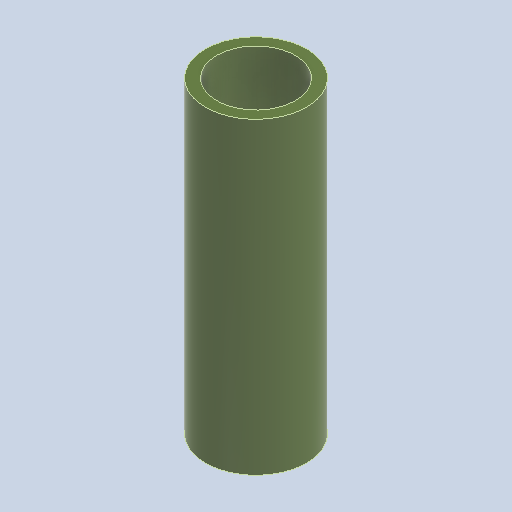
# Autodesk Inventor part: rotor_sleeve
Saved by Autodesk Inventor 2025 (Build 290162000, 162)
## iProperties
Created: 2026-08-13
Part Number: rotor_sleeve
Material: Ogólny
Document SubType Name: Modeling
Designer: zzapa
Density: 1 g/cm^3
Appearance: Ciemnooliwkowa
Author: zzapa
Autodesk Inventor part; units mm, degrees
ref_plane "YZ Plane" through (0, 0, 0) normal (1, 0, 0) x (0, 1, 0)
ref_plane "XZ Plane" through (0, 0, 0) normal (0, 1, 0) x (-1, 0, 0)
ref_plane "XY Plane" through (0, 0, 0) normal (0, 0, 1) x (1, 0, 0)
sketch "Szkic1" plane through (0, 0, 0) normal (0, 1, 0) x (-1, 0, 0)
  circle A0 centre (0, 0) radius 5.25
  circle A1 centre (0, 0) radius 4.075
  dimension "d0" = 8.15
  dimension "d1" = 10.5
  constraints: 2 centre point, 2 coincident
  measures "d0" diameter of A1
  measures "d1" diameter of A0
extrude "Wyciągnięcie proste1" add sketch "Szkic1" along normal blind 32
equation "\"d0\" = rotor_sleeve_in_D"
equation "\"d1\" = rotor_sleeve_out_D"
equation "\"d2\" = rotor_sleeve_h"
equation "\"insert_m2_d\" = 2.9"
equation "\"insert_m2_h\" = 7"
equation "\"insert_m2_corner\" = 0.5"
equation "\"insert_m2_pocket_d\" = 2.6"
equation "\"insert_m2_pocket_D\" = 4.5"
equation "\"insert_m2_pocket_nut_h\" = 1.5"
equation "\"stator_r_out\" = 30.15"
equation "\"stator_out_d\" = 3.2"
equation "\"stator_h\" = 45"
equation "\"stator_radial_screw_d\" = 4"
equation "\"stator_radial_screw_pos\" = 4"
equation "\"mag_size_x\" = 7"
equation "\"mag_size_y\" = 3"
equation "\"mag_corner_r\" = 0.4"
equation "\"magnet_ring_r\" = 26.95"
equation "\"magnet_ring_d\" = 3.3"
equation "\"magnet_ring_h\" = 36"
equation "\"magnet_ring_pocket_mag_size_x\" = 7.1"
equation "\"magnet_ring_pocket_mag_size_y\" = 3.1"
equation "\"magnet_ring_pocket_mag_size_z\" = 10.1"
equation "\"magnet_ring_pocket_radial_cut\" = 1.4"
equation "\"magnet_ring_insert_part_lengthen\" = 8"
equation "\"magnet_ring_insert_part_axial_flat_cut\" = 0.17"
equation "\"magnet_ring_insert_pos\" = 4"
equation "\"casing_d\" = 3"
equation "\"casing_r_in\" = 30.15"
equation "\"casing_lock_hole_r\" = 14.25"
equation "\"casing_lock_h\" = 8"
equation "\"casing_stator_fix_r\" = 23"
equation "\"casing_stator_fix_h\" = 6"
equation "\"casing_sidebar_length\" = 3"
equation "\"casing_vent_hole_length\" = 4"
equation "\"casing_vent_hole_width\" = 6"
equation "\"casing_head_insert_r\" = 19"
equation "\"casing_radial_stator_insert_pos\" = 18.1"
equation "\"rotor_out_r\" = 22.5"
equation "\"rotor_coil_groove_in_r\" = 17"
equation "\"rotor_coil_groove_ang\" = 18deg"
equation "\"rotor_core_r\" = 14.97"
equation "\"rotor_coil_groove_in_correction_r\" = 18"
equation "\"rotor_plastic_h\" = 32"
equation "\"rotor_teeth_d\" = 1.5"
equation "\"rotor_plastic_insert_r\" = 37"
equation "\"shaft_d\" = 8"
equation "\"shaft_lock_1_d\" = 8.1"
equation "\"shaft_lock_1_D\" = 44"
equation "\"shaft_lock_1_h1\" = 3.5"
equation "\"shaft_lock_1_corner\" = 2"
equation "\"shaft_lock_1_rotor_insert_grove_d_in\" = 36"
equation "\"shaft_lock_1_rotor_insert_grove_width_out\" = 5.5"
equation "\"shaft_lock_1_rotor_insert_grove_width_in\" = 7.6"
equation "\"shaft_lock_1_rotor_insert_r\" = 37"
equation "\"shaft_lock_1_shaft_insert_axial_cut_out_width\" = 12"
equation "\"shaft_lock_1_shaft_insert_axial_cut_in_width\" = 5.4"
equation "\"shaft_lock_1_shaft_insert_pos\" = 2.5"
equation "\"shaft_lock_1_shaft_insert_corner\" = 2"
equation "\"shaft_lock_1_shaft_insert_corner_finish\" = 0.5"
equation "\"shaft_lock_2_d\" = 8.1"
equation "\"shaft_lock_2_D\" = 44"
equation "\"shaft_lock_2_h1\" = 3.5"
equation "\"shaft_lock_2_corner\" = 2"
equation "\"shaft_lock_2_rotor_insert_grove_d_in\" = 36"
equation "\"shaft_lock_2_rotor_insert_grove_width_out\" = 5.5"
equation "\"shaft_lock_2_rotor_insert_grove_width_in\" = 7.6"
equation "\"shaft_lock_2_rotor_insert_r\" = 37"
equation "\"shaft_lock_2_shaft_insert_axial_cut_out_width\" = 12"
equation "\"shaft_lock_2_shaft_insert_axial_cut_in_width\" = 5.4"
equation "\"shaft_lock_2_shaft_insert_pos\" = 2.5"
equation "\"shaft_lock_2_shaft_insert_corner\" = 2"
equation "\"shaft_lock_2_shaft_insert_corner_finish\" = 0.5"
equation "\"commutator_plastic_shaft_d\" = 8.1"
equation "\"commutator_plastic_h\" = 17"
equation "\"commutator_plastic_insert_cut_deepness\" = 0.5"
equation "\"commutator_plastic_insert_cut_length\" = 6"
equation "\"commutator_plastic_insert_pos\" = 3"
equation "\"commutator_plate_D\" = 22"
equation "\"commutator_plate_d\" = 1"
equation "\"commutator_plate_ang\" = 55deg"
equation "\"commutator_plate_h\" = 17"
equation "\"commutator_plate_insert_pos\" = 3"
equation "\"sleeve_in_r\" = 11.1"
equation "\"sleeve_d\" = 3"
equation "\"sleeve_h\" = 7"
equation "\"sleeve_cup_r\" = 22"
equation "\"sleeve_cup_h\" = 4.5"
equation "\"sleeve_head_insert_r\" = 19"
equation "\"rotor_sleeve_out_D\" = 10.5"
equation "\"rotor_sleeve_in_D\" = 8.15"
equation "\"rotor_sleeve_h\" = 32"
equation "\"carbon_brush_batt_h\" = 8"
equation "\"carbon_brush_batt_d\" = 4"
equation "\"brush_cart_outer_holder_width\" = 5.5"
equation "\"brush_cart_outer_holder_arc_r\" = 33.15"
equation "\"brush_cart_outer_holder_arc_pos\" = 1.5"
equation "\"casing_cart_hole_corner\" = 1"
equation "\"casing_cart_hole_width\" = 2.6"
equation "\"casing_cart_hole_ang\" = 90deg"
equation "\"brush_holder_batt_arc_r\" = 30.15"
equation "\"brush_holder_batt_width\" = 16"
equation "\"brush_holder_batt_insert_flat_length\" = 6"
equation "\"brush_holder_batt_insert_flat_depth\" = 6"
equation "\"brush_holder_batt_insert_flat_width\" = 2"
equation "\"brush_holder_batt_brush_hole_d\" = 4.5"
equation "\"casing_backsleeve_insert_pos\" = 4.9"
equation "\"casing_cart_hole_pos\" = 17"
equation "\"casing_sleeve_cut_d\" = 46"
equation "\"casing_sleeve_cut_h\" = 4"
equation "\"name_plate_D\" = 45"
equation "\"name_plate_d\" = 28"
equation "\"name_plate_insert_r\" = 19"
equation "\"sleeve_bearing_material_lock_h\" = 2"
equation "\"back_sleeve_D\" = 66"
equation "\"back_sleeve_d\" = 22.2"
equation "\"back_sleeve_h\" = 5"
equation "\"commutator_back_plate_lock_h\" = 2"
equation "\"commutator_back_plate_lock_r\" = 23"
equation "\"commutator_plastic_back_plate_lock_r\" = 11.9"
equation "\"commutator_plastic_back_plate_lock_h\" = 1"
equation "\"commutator_plastic_back_plate_hook_in_r\" = 11.15"
equation "\"commutator_plastic_back_plate_hook_d\" = 1"
